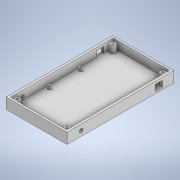
# Autodesk Inventor part: pudelko dol
Saved by Autodesk Inventor 2022 (Build 260153000, 153)
## iProperties
Created: 2022-04-02
Part Number: pudelko dol
Material: Ogólny
Document SubType Name: Modeling
Designer: jolow
Density: 1 g/cm^3
Appearance: Domyślna
Author: jolow
Autodesk Inventor part; units mm, degrees
ref_plane "YZ Plane" through (0, 0, 0) normal (1, 0, 0) x (0, 1, 0)
ref_plane "XZ Plane" through (0, 0, 0) normal (0, 1, 0) x (-1, 0, 0)
ref_plane "XY Plane" through (0, 0, 0) normal (0, 0, 1) x (1, 0, 0)
sketch "Szkic1" plane through (0, 0, 0) normal (0, 1, 0) x (-1, 0, 0)
  line L0 (0, 0) -> (102.05, 0)
  line L1 (102.05, 0) -> (102.05, 178.85)
  line L2 (102.05, 178.85) -> (0, 178.85)
  line L3 (0, 178.85) -> (0, 0)
  dimension "d0" = 178.85
  dimension "d1" = 102.05
  constraints: 8 end point, 2 parallel, 1 horizontal, 1 perpendicular
  measures "d0" distance of L0.end L1.end
  measures "d1" distance of L1.end L2.end
extrude "Wyciągnięcie proste1" add sketch "Szkic1" along normal blind 17.75
sketch "Szkic2" plane through (0, 17.75, 0) normal (0, 1, 0) x (1, 0, 0)
  line L0 (-98.1, -3.35) -> (-3.95, -3.35)
  line L1 (-3.95, -3.35) -> (-3.95, -175.5)
  line L2 (-3.95, -175.5) -> (-98.1, -175.5)
  line L3 (-98.1, -175.5) -> (-98.1, -3.35)
  line L4 (-102.05, -178.85) -> (0, -178.85) projected
  line L5 (0, 0) -> (-102.05, 0) projected
  line L6 (-102.05, 0) -> (-102.05, -178.85) projected
  line L7 (0, -178.85) -> (0, 0) projected
  dimension "d4" = 3.35
  dimension "d5" = 3.35
  dimension "d6" = 3.95
  dimension "d7" = 3.95
  constraints: 8 end point, 2 parallel, 1 horizontal, 1 perpendicular
  measures "d4" distance between parallel lines of L4 L2
  measures "d5" distance between parallel lines of L5 L0
  measures "d6" distance between parallel lines of L6 L3
  measures "d7" distance between parallel lines of L7 L1
extrude "Wyciągnięcie proste2" cut sketch "Szkic2" against normal blind 14.35 contours L0 L1 L2 L3
sketch "Szkic3" plane through (0, 3.4, 0) normal (0, 1, 0) x (1, 0, 0)
  circle A0 centre (-9.4, -9.45) radius 4.375
  circle A1 centre (-92.65, -9.45) radius 4.375
  circle A2 centre (-92.5, -63.1) radius 3
  circle A3 centre (-9.3, -62.65) radius 3
  circle A4 centre (-92.4, -115.4999) radius 3
  circle A5 centre (-9.05, -115.7994) radius 3
  circle A6 centre (-92.35, -169.9) radius 4.375
  circle A7 centre (-8.9504, -170.15) radius 4.375
  line L0 (-102.05, 0) -> (-102.05, -178.85) projected
  line L1 (0, 0) -> (-102.05, 0) projected
  line L2 (0, -178.85) -> (0, 0) projected
  line L3 (-98.1, -175.5) -> (-98.1, -3.35) projected
  line L4 (-3.95, -3.35) -> (-3.95, -175.5) projected
  dimension "d10" = 8.75
  dimension "d11" = 8.75
  dimension "d12" = 6
  dimension "d13" = 6
  dimension "d14" = 6
  dimension "d15" = 6
  dimension "d16" = 8.75
  dimension "d17" = 8.75
  dimension "d18" = 9.4
  dimension "d19" = 9.45
  dimension "d20" = 9.45
  dimension "d21" = 9.4
  dimension "d23" = 63.1
  dimension "d25" = 62.65
  dimension "d27" = 52.4
  dimension "d29" = 53.15
  dimension "d30" = 83.2
  dimension "d31" = 102.05
  dimension "d32" = 9.55
  dimension "d33" = 9.65
  dimension "d34" = 83.35
  dimension "d35" = 83.4
  dimension "d36" = 9.7
  dimension "d37" = 160.45
  dimension "d38" = 160.7
  constraints: 8 centre point
  measures "d10" diameter of A1
  measures "d11" diameter of A0
  measures "d12" diameter of A2
  measures "d13" diameter of A3
  measures "d14" diameter of A5
  measures "d15" diameter of A4
  measures "d16" diameter of A6
  measures "d17" diameter of A7
  measures "d18" distance from line of L0 A1.centre
  measures "d19" distance from line of L1 A1.centre
  measures "d20" distance from line of L1 A0.centre
  measures "d21" distance from line of L2 A0.centre
  measures "d23" distance from line of L1 A2.centre
  measures "d25" distance from line of L1 A3.centre
  measures "d27" distance of A2.centre A4.centre
  measures "d29" distance of A3.centre A5.centre
  measures "d30" horizontal distance of A2.centre A3.centre
  measures "d31" distance of L1.start L0.start
  measures "d32" distance from line of L0 A2.centre
  measures "d33" distance from line of L0 A4.centre
  measures "d34" horizontal distance of A5.centre A4.centre
  measures "d35" distance of A7.centre A6.centre
  measures "d36" distance from line of L0 A6.centre
  measures "d37" distance of A1.centre A6.centre
  measures "d38" vertical distance of A0.centre A7.centre
extrude "Wyciągnięcie proste3" add sketch "Szkic3" along normal blind 12 contours A0 | A1 | A6 | A7
sketch "Szkic4" plane through (-0.0028, 3.4, -0.0047) normal (0, 1, 0) x (1, 0, 0)
  circle A0 centre (-9.4, -9.45) radius 4.375
  circle A1 centre (-92.65, -9.45) radius 4.375
  circle A2 centre (-92.5, -63.1) radius 3
  circle A3 centre (-9.3, -62.65) radius 3
  circle A4 centre (-92.4, -115.4999) radius 3
  circle A5 centre (-9.05, -115.7994) radius 3
  circle A6 centre (-92.35, -169.9) radius 4.375
  circle A7 centre (-8.9504, -170.15) radius 4.375
  line L0 (-102.05, 0) -> (-102.05, -178.85)
  line L1 (0, 0) -> (-102.05, 0)
  line L2 (0, -178.85) -> (0, 0)
  line L3 (-98.1, -175.5) -> (-98.1, -3.35)
  line L4 (-3.95, -3.35) -> (-3.95, -175.5)
  dimension "d59" = 8.75
  dimension "d62" = 8.75
  dimension "d56" = 6
  dimension "d53" = 6
  dimension "d47" = 6
  dimension "d50" = 6
  dimension "d44" = 8.75
  dimension "d41" = 8.75
  dimension "d61" = 9.4
  dimension "d60" = 9.45
  dimension "d64" = 9.45
  dimension "d63" = 9.4
  dimension "d58" = 63.1
  dimension "d55" = 62.65
  dimension "d52" = 52.4
  dimension "d49" = 53.15
  dimension "d54" = 83.2
  dimension "d68" = 102.05
  dimension "d57" = 9.55
  dimension "d51" = 9.65
  dimension "d48" = 83.35
  dimension "d43" = 83.4
  dimension "d46" = 9.7
  dimension "d45" = 160.45
  dimension "d42" = 160.7
  constraints: 10 end point, 8 centre point
  measures "d59" diameter of A1
  measures "d62" diameter of A0
  measures "d56" diameter of A2
  measures "d53" diameter of A3
  measures "d47" diameter of A5
  measures "d50" diameter of A4
  measures "d44" diameter of A6
  measures "d41" diameter of A7
  measures "d61" distance from line of L0 A1.centre
  measures "d60" distance from line of L1 A1.centre
  measures "d64" distance from line of L1 A0.centre
  measures "d63" distance from line of L2 A0.centre
  measures "d58" distance from line of L1 A2.centre
  measures "d55" distance from line of L1 A3.centre
  measures "d52" distance of A2.centre A4.centre
  measures "d49" distance of A3.centre A5.centre
  measures "d54" horizontal distance of A2.centre A3.centre
  measures "d68" distance of L1.start L0.start
  measures "d57" distance from line of L0 A2.centre
  measures "d51" distance from line of L0 A4.centre
  measures "d48" horizontal distance of A5.centre A4.centre
  measures "d43" distance of A7.centre A6.centre
  measures "d46" distance from line of L0 A6.centre
  measures "d45" distance of A1.centre A6.centre
  measures "d42" vertical distance of A0.centre A7.centre
extrude "Wyciągnięcie proste4" add sketch "Szkic4" along normal blind 4.9 contours A2 | A3 | A4 | A5
sketch "Szkic5" plane through (-92.65, 15.4, 9.45) normal (0, 1, 0) x (1, 0, 0)
  circle A0 centre (0, 0) radius 1.975
  circle A1 centre (83.25, 0) radius 4.375 projected
  circle A2 centre (83.25, 0) radius 1.975
  circle A3 centre (0.1472, -53.6453) radius 3 projected
  circle A4 centre (0.1472, -53.6453) radius 1.2
  circle A5 centre (83.3472, -53.1953) radius 3 projected
  circle A6 centre (83.3472, -53.1953) radius 1.2
  circle A7 centre (0.2472, -106.0452) radius 3 projected
  circle A8 centre (0.2472, -106.0452) radius 1.2
  circle A9 centre (83.5972, -106.3447) radius 3 projected
  circle A10 centre (83.5972, -106.3447) radius 1.2
  circle A11 centre (0.3, -160.45) radius 4.375 projected
  circle A12 centre (0.3, -160.45) radius 1.975
  circle A13 centre (83.6996, -160.7) radius 4.375 projected
  circle A14 centre (83.6996, -160.7) radius 1.975
  point P0 (92.65, 9.45)
  dimension "d69" = 3.95
  dimension "d70" = 3.95
  dimension "d71" = 2.4
  dimension "d72" = 2.4
  dimension "d73" = 2.4
  dimension "d74" = 2.4
  dimension "d75" = 3.95
  dimension "d76" = 3.95
  constraints: 8 centre point, 7 coincident
  measures "d69" diameter of A0
  measures "d70" diameter of A2
  measures "d71" diameter of A4
  measures "d72" diameter of A6
  measures "d73" diameter of A8
  measures "d74" diameter of A10
  measures "d75" diameter of A14
  measures "d76" diameter of A12
extrude "Wyciągnięcie proste5" cut sketch "Szkic5" against normal through all contours A0 | A2 | A4 | A6 | A8 | A10 | A12 | A14
sketch "Szkic6" plane through (-98.1, 17.75, 175.5) normal (1, 0, 0) x (0, 0, -1)
  line L0 (144.273, -4.35) -> (156.273, -4.35)
  line L1 (156.273, -4.35) -> (156.273, -14.35)
  line L2 (156.273, -14.35) -> (144.273, -14.35)
  line L3 (144.273, -14.35) -> (144.273, -4.35)
  line L4 (0, -14.35) -> (172.15, -14.35) projected
  point P0 (175.5, -17.75)
  dimension "d79" = 10
  dimension "d80" = 12
  constraints: 8 end point, 2 parallel, 1 collinear, 1 horizontal, 1 perpendicular
  measures "d79" distance of L0.end L1.end
  measures "d80" distance of L0.start L0.end
extrude "Wyciągnięcie proste6" cut sketch "Szkic6" along normal through all both and the other way through all
sketch "Szkic7" plane through (-102.05, 0, 0) normal (-1, 0, 0) x (0, 0, 1)
  circle A0 centre (155.3753, 8.4) radius 3
  line L0 (19.227, 3.4) -> (19.227, 13.4) projected
  point P0 (0, 0)
  point P1 (19.227, 8.4)
  dimension "d83" = 6
  constraints: 1 centre point, 1 horizontal alignment, 1 midpoint
  measures "d83" diameter of A0
extrude "Wyciągnięcie proste7" cut sketch "Szkic7" along normal through all both and the other way through all
